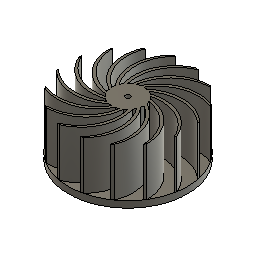
Tunnel (Autodesk Fusion 360 archive; units mm, degrees)
design "helice"
Autodesk Fusion 360 part; units mm, degrees
sketch "Sketch1" plane through (0, 0, 0) normal (0, 1, 0) x (1, 0, 0)
  circle A0 centre (0, 0) radius 5
  circle A1 centre (0, 0) radius 18.5
  circle A2 centre (0, 0) radius 0.75
  line L0 (-21, 0) -> (20.3872, 0) construction
  line L1 (0, 20) -> (0, -20) construction
  arc A3 (10.124, -15.484) -> (5, 0) centre (-1.6517, -10.791) ccw
  arc A4 (15.2788, -10.4311) -> (4.6194, 1.9134) centre (2.6036, -10.6017) ccw
  arc A5 (18.1076, -3.7901) -> (3.5355, 3.5355) centre (6.4625, -8.7984) ccw
  arc A6 (18.1796, 3.4279) -> (1.9134, 4.6194) centre (9.3375, -5.6555) ccw
  arc A7 (15.484, 10.124) -> (0, 5) centre (10.791, -1.6517) ccw
  arc A8 (10.4311, 15.2788) -> (-1.9134, 4.6194) centre (10.6017, 2.6036) ccw
  arc A9 (3.7901, 18.1076) -> (-3.5355, 3.5355) centre (8.7984, 6.4625) ccw
  arc A10 (-3.4279, 18.1796) -> (-4.6194, 1.9134) centre (5.6555, 9.3375) ccw
  arc A11 (-10.124, 15.484) -> (-5, 0) centre (1.6517, 10.791) ccw
  arc A12 (-15.2788, 10.4311) -> (-4.6194, -1.9134) centre (-2.6036, 10.6017) ccw
  arc A13 (-18.1076, 3.7901) -> (-3.5355, -3.5355) centre (-6.4625, 8.7984) ccw
  arc A14 (-18.1796, -3.4279) -> (-1.9134, -4.6194) centre (-9.3375, 5.6555) ccw
  arc A15 (-15.484, -10.124) -> (0, -5) centre (-10.791, 1.6517) ccw
  arc A16 (-10.4311, -15.2788) -> (1.9134, -4.6194) centre (-10.6017, -2.6036) ccw
  arc A17 (-3.7901, -18.1076) -> (3.5355, -3.5355) centre (-8.7984, -6.4625) ccw
  arc A18 (3.4279, -18.1796) -> (4.6194, -1.9134) centre (-5.6555, -9.3375) ccw
  arc A19 (10.7478, -15.0577) -> (4.9076, 0.9567) centre (-0.8522, -10.2159) ccw
  line L2 (10.7478, -15.0577) -> (10.124, -15.484)
  arc A20 (15.692, -9.7985) -> (4.168, 2.7619) centre (3.1221, -9.7644) ccw
  line L3 (15.692, -9.7985) -> (15.2788, -10.4311)
  arc A21 (18.2472, -3.0476) -> (2.7938, 4.1467) centre (6.6211, -7.8264) ccw
  line L4 (18.2472, -3.0476) -> (18.1076, -3.7901)
  arc A22 (18.0245, 4.1673) -> (0.9942, 4.9002) centre (9.1122, -4.6968) ccw
  line L5 (18.0245, 4.1673) -> (18.1796, 3.4279)
  arc A23 (15.0577, 10.7478) -> (-0.9567, 4.9076) centre (10.2159, -0.8522) ccw
  line L6 (15.0577, 10.7478) -> (15.484, 10.124)
  arc A24 (9.7985, 15.692) -> (-2.7619, 4.168) centre (9.7644, 3.1221) ccw
  line L7 (9.7985, 15.692) -> (10.4311, 15.2788)
  arc A25 (3.0476, 18.2472) -> (-4.1467, 2.7938) centre (7.8264, 6.6211) ccw
  line L8 (3.0476, 18.2472) -> (3.7901, 18.1076)
  arc A26 (-4.1673, 18.0245) -> (-4.9002, 0.9942) centre (4.6968, 9.1122) ccw
  line L9 (-4.1673, 18.0245) -> (-3.4279, 18.1796)
  arc A27 (-10.7478, 15.0577) -> (-4.9076, -0.9567) centre (0.8522, 10.2159) ccw
  line L10 (-10.7478, 15.0577) -> (-10.124, 15.484)
  arc A28 (-15.692, 9.7985) -> (-4.168, -2.7619) centre (-3.1221, 9.7644) ccw
  line L11 (-15.692, 9.7985) -> (-15.2788, 10.4311)
  arc A29 (-18.2472, 3.0476) -> (-2.7938, -4.1467) centre (-6.6211, 7.8264) ccw
  line L12 (-18.2472, 3.0476) -> (-18.1076, 3.7901)
  arc A30 (-18.0245, -4.1673) -> (-0.9942, -4.9002) centre (-9.1122, 4.6968) ccw
  line L13 (-18.0245, -4.1673) -> (-18.1796, -3.4279)
  arc A31 (-15.0577, -10.7478) -> (0.9567, -4.9076) centre (-10.2159, 0.8522) ccw
  line L14 (-15.0577, -10.7478) -> (-15.484, -10.124)
  arc A32 (-9.7985, -15.692) -> (2.7619, -4.168) centre (-9.7644, -3.1221) ccw
  line L15 (-9.7985, -15.692) -> (-10.4311, -15.2788)
  arc A33 (-3.0476, -18.2472) -> (4.1467, -2.7938) centre (-7.8264, -6.6211) ccw
  line L16 (-3.0476, -18.2472) -> (-3.7901, -18.1076)
  arc A34 (4.1673, -18.0245) -> (4.9002, -0.9942) centre (-4.6968, -9.1122) ccw
  line L17 (4.1673, -18.0245) -> (3.4279, -18.1796)
  dimension "d1" = 10
  dimension "d2" = 37
  dimension "d3" = 1.5
  dimension "d5" = 360
  dimension "d7" = 360
  constraint coincident A0.centre A1.centre
  constraint concentric A0 A1
  constraint concentric A1 A2
  constraint horizontal L0
  constraint vertical L1
  constraint coincident A1 A3.start
  constraint coincident A0 A3.end
  constraint coincident L0 A3.end
  constraint coincident A1 A19.start
  constraint coincident A0 A19.end
  measures "d1" diameter of A0
  measures "d2" diameter of A1
  measures "d3" diameter of A2
extrude "Extrude2" add sketch "Sketch1" against normal blind 2 contours A0 | A0 A1 A3 A34 | A0 A3 A19 L2 | A0 A1 A4 A19 | A0 A18 A34 L17 | A1 L2 | A0 A4 A20 L3 | A0 A1 A18 A33 | A1 L17 | A0 A1 A5 A20 | A1 L3 | A0 A17 A33 L16 | A0 A5 A21 L4 | A0 A1 A17 A32 | A1 L16 | A0 A1 A6 A21 | A1 L4 | A0 A16 A32 L15 | A0 A6 A22 L5 | A0 A1 A16 A31 | A1 L15 | A0 A1 A7 A22 | A1 L5 | A0 A15 A31 L14 | A0 A7 A23 L6 | A0 A1 A15 A30 | A1 L14 | A0 A1 A8 A23 | A1 L6 | A0 A14 A30 L13 | A0 A8 A24 L7 | A0 A1 A14 A29 | A1 L13 | A0 A1 A9 A24 | A1 L7 | A0 A13 A29 L12 | A0 A9 A25 L8 | A0 A1 A13 A28 | A1 L12 | A0 A1 A10 A25 | A1 L8 | A0 A12 A28 L11 | A0 A10 A26 L9 | A0 A1 A12 A27 | A1 L11 | A0 A1 A11 A26 | A1 L9 | A0 A11 A27 L10 | A1 L10 | A2 makes body 1
extrude "Extrude1" add sketch "Sketch1" along normal blind 15 separate body contours A0 | A0 A3 A19 L2 | A0 A18 A34 L17 | A0 A4 A20 L3 | A0 A17 A33 L16 | A0 A5 A21 L4 | A0 A16 A32 L15 | A0 A6 A22 L5 | A0 A15 A31 L14 | A0 A7 A23 L6 | A0 A14 A30 L13 | A0 A8 A24 L7 | A0 A13 A29 L12 | A0 A9 A25 L8 | A0 A12 A28 L11 | A0 A10 A26 L9 | A0 A11 A27 L10 makes body 2
extrude "Extrude3" cut sketch "Sketch1" against normal blind 2 contours A2 bodies 1

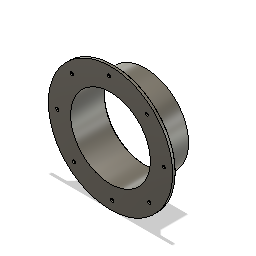
design "Bague d'adaptation tunnel"
Autodesk Fusion 360 part; units mm, degrees
sketch "Sketch1" plane through (0, 0, 0) normal (0, 1, 0) x (1, 0, 0)
  line L0 (0, 0) -> (-35, 0)
  line L1 (-35, 0) -> (-35, 5)
  line L2 (-35, 5) -> (-5, 5)
  line L3 (-5, 5) -> (-5, 55)
  line L4 (-5, 55) -> (0, 55)
  line L5 (0, 55) -> (0, 0)
  line L6 (62.5, 0) -> (62.5, 74.9074) construction
  dimension "d1" = 35
  dimension "d2" = 62.5
  dimension "d12" = 5
  dimension "d13" = 5
  constraint coincident L0.start L5.end
  constraint horizontal L0
  constraint perpendicular L0 L1
  constraint perpendicular L1 L2
  constraint perpendicular L2 L3
  constraint perpendicular L3 L4
  constraint perpendicular L0 L5
  constraint vertical L6
  measures "d1" distance of L0.start L0.end
  measures "d2" distance of L5 L6
  measures "d12" distance of L0 L2
  measures "d13" distance of L3 L5
revolve "Revolve1" add sketch "Sketch1" angle 360 about axis through (62.5, 0, 0) along (0, 0, -1)
sketch "Sketch2" plane through (0, 0, 0) normal (0, 0, 1) x (1, 0, 0)
sketch "Sketch3" plane through (0, 0, -5) normal (0, 0, -1) x (-1, 0, 0)
  circle A0 centre (-62.5, 0) radius 97.5
  circle A1 centre (-62.5, 0) radius 67.5
sketch "Sketch4" plane through (0, 0, -5) normal (0, 0, -1) x (1, 0, 0)
sketch "Sketch5" plane through (0, 0, -5) normal (0, 0, -1) x (1, 0, 0)
sketch "Sketch6" plane through (0, 0, 0) normal (0, 0, 1) x (1, 0, 0)
sketch "Sketch7" plane through (0, 0, -5) normal (0, 0, -1) x (1, 0, 0)
  line L0 (65, 68.5) -> (65, 98.5) construction
  circle A0 centre (65, 83.5) radius 2.5
  dimension "d5" = 5
  constraint vertical L0
  constraint midpoint L0 A0.centre
  measures "d5" diameter of A0
extrude "Extrude1" cut sketch "Sketch7" against normal up to surface (5 mm away)
chamfer "Chamfer1" distance 3 angle 45 1 edges at (62.6692, -84.404, -5)
pattern_circular "C-Pattern1" count 8 over 360 about axis through (62.5, 0, 55) along (0, 0, -1) of 2 faces at (67.4876, -83.2511, -1.3333) (60.3814, -84.9246, -4.3333)
chamfer "Chamfer2" distance 2 angle 45 1 edges at (4.2295, 22.601, -55)
chamfer "Chamfer3" distance 1 angle 45 1 edges at (-28.4019, 35.2575, -5)
chamfer "Chamfer4" distance 7 angle 45 1 edges at (-0.4321, 24.409, -5)
equation "d2 = diamètre / 2"
equation "diamètre = 125 mm"
equation "epaisseur = 5 mm"
equation "d12 = epaisseur"
equation "d13 = epaisseur"

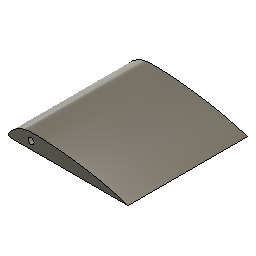
design "Profil_D"
Autodesk Fusion 360 part; units mm, degrees
sketch "Sketch2" plane through (0, 0, 0) normal (0, 0, 1) x (1, 0, 0)
  spline S0 degree 5 poles (-150, -30) (-148.6317, -27.6875) (-145.7466, -23.1113) (-140.9734, -16.3936) (-133.7178, -7.7297) (-123.2027, 2.588) (-111.3696, 12.323) (-98.4739, 21.3377) (-84.9516, 29.3984) (-71.442, 36.1708) (-58.6129, 41.3677) (-46.994, 44.8998) (-36.8317, 46.9886) (-27.8889, 48.4044) (-18.8428, 49.4447) (-8.1843, 50.2071) (5.0951, 50.6844) (20.9364, 50.8977) (38.6438, 50.8689) (57.1451, 50.6259) (75.3307, 50.1948) (92.3315, 49.5973) (107.8928, 48.8453) (122.3003, 47.9423) (136.1425, 46.8868) (150.1203, 45.6746) (164.853, 44.3022) (180.6465, 42.7694) (197.5028, 41.08) (215.2286, 39.2403) (233.5104, 37.2587) (252.0045, 35.1445) (270.4181, 32.9074) (288.5997, 30.5563) (306.5028, 28.1005) (324.1447, 25.55) (341.5675, 22.9164) (358.7974, 20.2137) (375.8064, 17.4592) (392.4679, 14.6742) (408.6088, 11.8782) (424.0662, 9.0834) (438.747, 6.2875) (452.676, 3.4691) (466.0736, 0.5783) (479.3235, -2.4561) (492.8525, -5.707) (507.0324, -9.232) (522.0804, -13.0571) (537.94, -17.1558) (554.3317, -21.4602) (570.8401, -25.8774) (586.9902, -30.3049) (602.3236, -34.6454) (616.4851, -38.8241) (629.271, -42.7978) (638.3173, -45.7955) (644.4227, -47.9386) (648.1912, -49.3206) (650, -50) knots 0 0 0 0 0 0 0.018182 0.036364 0.054545 0.072727 0.090909 0.109091 0.127273 0.145455 0.163636 0.181818 0.2 0.218182 0.236364 0.254545 0.272727 0.290909 0.309091 0.327273 0.345455 0.363636 0.381818 0.4 0.418182 0.436364 0.454545 0.472727 0.490909 0.509091 0.527273 0.545455 0.563636 0.581818 0.6 0.618182 0.636364 0.654545 0.672727 0.690909 0.709091 0.727273 0.745455 0.763636 0.781818 0.8 0.818182 0.836364 0.854545 0.872727 0.890909 0.909091 0.927273 0.945455 0.963636 0.981818 1 1 1 1 1 1
  spline S1 degree 5 poles (-150, -30) (-150.2907, -30.9013) (-150.7689, -32.5877) (-151.1775, -34.7724) (-151.0973, -36.9606) (-150.1199, -39.2209) (-148.5514, -42.2733) (-146.0589, -45.3385) (-142.8997, -47.6377) (-139.9521, -49.1653) (-136.4539, -50.0554) (-130.6576, -50.5032) (-121.4836, -50.661) (-108.4255, -50.6441) (-91.4444, -50.5352) (-70.8621, -50.3905) (-47.2573, -50.2442) (-21.3618, -50.1142) (6.043, -50.0071) (34.226, -49.9229) (62.6177, -49.8607) (90.8045, -49.8192) (118.5062, -49.7967) (145.5601, -49.7909) (171.9023, -49.7996) (197.5513, -49.8202) (222.591, -49.85) (247.1538, -49.8864) (271.4045, -49.9268) (295.5238, -49.9686) (319.6923, -50.0096) (344.0732, -50.0479) (368.7998, -50.0818) (393.9804, -50.11) (419.7003, -50.1316) (446.0253, -50.1455) (473.004, -50.1514) (500.6704, -50.1488) (529.0468, -50.1375) (558.1461, -50.1172) (587.974, -50.0879) (612.4201, -50.0572) (631.0827, -50.0302) (643.67, -50.0104) (650, -50) knots 0 0 0 0 0 0 0.025 0.05 0.075 0.1 0.125 0.15 0.175 0.2 0.225 0.25 0.275 0.3 0.325 0.35 0.375 0.4 0.425 0.45 0.475 0.5 0.525 0.55 0.575 0.6 0.625 0.65 0.675 0.7 0.725 0.75 0.775 0.8 0.825 0.85 0.875 0.9 0.925 0.95 0.975 1 1 1 1 1 1
  circle A0 centre (0, 0) radius 19.9529
  line L0 (-112.409, 30.2253) -> (27.8025, 61.2999)
  point P0 (-100, 20)
  point P1 (-42.3033, 45.7626)
  point P2 (-10, 50)
  point P3 (80, 50)
  point P4 (154.5456, 45.25)
  point P5 (252.9701, 34.9974)
  point P6 (360, 20)
  point P7 (445, 5)
  point P8 (510, -10)
  point P9 (597.5872, -33.3286)
  point P10 (-151, -36)
  point P11 (-150, -39.3322)
  point P12 (-147, -44)
  point P13 (-142, -48)
  point P14 (-135.4793, -50)
  point P15 (10.0145, -50)
  point P16 (314.2802, -50)
  constraint coincident A0.centre origin
  constraint midpoint P1 L0
extrude "Extrude1" add sketch "Sketch2" along normal blind 800
scale "Scale1" factor 0.1 about (-150, -30, 0) bodies 1
move_body "Move1" bodies 1 to x (1, 0, 0) y (0, 1, 0) z (0, 0, 1) at (135, 27, 0)

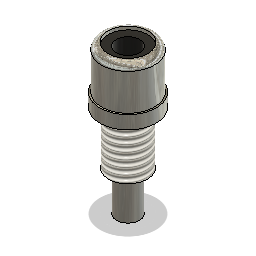
design "CINCH"
Autodesk Fusion 360 part; units mm, degrees
sketch "Sketch1" plane through (0, 0, 0) normal (0, 1, 0) x (1, 0, 0)
  circle A0 centre (0, 0) radius 3
  circle A1 centre (0, 0) radius 4
  circle A2 centre (0, 0) radius 4.25
  circle A3 centre (0, 0) radius 1.75
  dimension "d1" = 6
  dimension "d2" = 8
  dimension "d3" = 8.5
  dimension "d4" = 3.5
  constraint coincident A0.centre A1.centre
  constraint concentric A0 A1
  constraint concentric A0 A3
  measures "d1" diameter of A0
  measures "d2" diameter of A1
  measures "d3" diameter of A2
  measures "d4" diameter of A3
extrude "Extrude1" add sketch "Sketch1" along normal blind 8.5 contours A1 makes body 1
extrude "Extrude2" add sketch "Sketch1" along normal blind 2 contours A2 bodies 1
extrude "Extrude3" add sketch "Sketch1" against normal blind 8 separate body contours A0 makes body 2
extrude "Extrude4" add sketch "Sketch1" against normal blind 14 contours A3 bodies 2
thread "Thread1" "ISO Metric profile 6.0 M6x1 6g" major diameter 5.884 minor diameter 4.7435 pitch 1 angle 60 resizes the face on face at (2.9963, -5.3333, 0.1495) on bodies 2
extrude "Extrude5" add sketch "Sketch1" along normal blind 8 separate body contours A0 makes body 3
fillet "Fillet1" radius 1 1 edges at (-3.7293, 8.5, 1.4465) on bodies 1

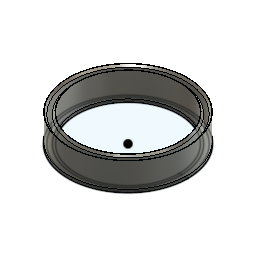
design "Capuchon de finition tunnel"
Autodesk Fusion 360 part; units mm, degrees
sketch "Sketch1" plane through (0, 0, 0) normal (0, 1, 0) x (1, 0, 0)
  circle A0 centre (0, 0) radius 62.5
  circle A1 centre (0, 0) radius 58.25
  circle A2 centre (0, 0) radius 65
  circle A3 centre (0, 0) radius 55.75
  dimension "d1" = 125
  dimension "d2" = 116.5
  dimension "d3" = 130
  dimension "d4" = 111.5
  constraint coincident A0.centre A1.centre
  constraint concentric A1 A2
  constraint concentric A1 A3
  measures "d1" diameter of A0 A1.centre
  measures "d2" diameter of A1 A0.centre
  measures "d3" diameter of A2
  measures "d4" diameter of A3
extrude "Extrude2" add sketch "Sketch1" along normal blind 30 makes body 1 at (64.677, 20, 6.4719) makes body 2 at (57.9605, 20, 5.7998)
extrude "Extrude1" add sketch "Sketch1" along normal blind 3 separate body contours A0 | A1 | A2 makes body 3
chamfer "Chamfer1" distance 2 angle 45 1 edges at (-54.3081, 30, 21.0641) on bodies 2
chamfer "Chamfer3" distance 2 angle 45 1 edges at (-58.2705, 30, -22.601) on bodies 1
sketch "Sketch2" plane through (0, 0, 0) normal (0, 1, 0) x (-1, 0, 0)

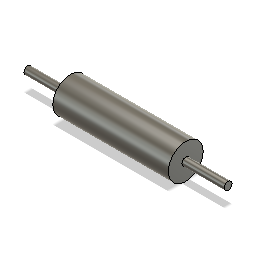
design "ResistancePuissance"
Autodesk Fusion 360 part; units mm, degrees
sketch "Sketch2" plane through (0, 0, 0) normal (1, 0, 0) x (0, 0, -1)
  circle A0 centre (0, 0) radius 2.25
  circle A1 centre (0, 0) radius 0.5
  dimension "d1" = 4.5
  dimension "d2" = 1
  constraint coincident A0.centre A1.centre
  constraint concentric A0 A1
  measures "d1" diameter of A0
  measures "d2" diameter of A1
extrude "Extrude1" add sketch "Sketch2" along normal mid plane 26 contours A1
extrude "Extrude2" add sketch "Sketch2" along normal mid plane 15
